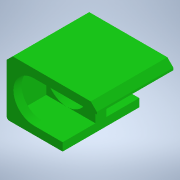
# Autodesk Inventor part: Y-linear bearing shroud secondary
Saved by Autodesk Inventor 2020 (Build 240168000, 168)
## iProperties
Created: 2021-02-25
Part Number: Y-linear bearing shroud secondary
Material: ABS Plastic
Document SubType Name: Modeling
Designer: AOB
Mass: 6.31823 g
Surface Area: 48.6976 cm^2
Volume: 5.96059 cm^3
Density: 1.06 g/cm^3
Appearance: Dark Green
Author: AOB
Autodesk Inventor part; units mm, degrees
ref_plane "YZ Plane" through (0, 0, 0) normal (1, 0, 0) x (0, 1, 0)
ref_plane "XZ Plane" through (0, 0, 0) normal (0, 1, 0) x (-1, 0, 0)
ref_plane "XY Plane" through (0, 0, 0) normal (0, 0, 1) x (1, 0, 0)
sketch "Sketch1" plane through (0, 0, 0) normal (0, 0, 1) x (1, 0, 0)
  line L0 (-9.0445, -10.4807) -> (0.0261, -10.458)
  line L1 (-10, 8.3388) -> (-10, 0)
  line L2 (-10, 0) -> (-9.9763, -9.4855)
  line L3 (-7.782, 10.5568) -> (20.782, 10.5568)
  line L4 (23, 8.3389) -> (23, 7.5575)
  line L5 (20.782, 10.5568) -> (23, 8.3389)
  line L6 (-7.782, 10.5568) -> (-10, 8.3388)
  arc A0 (-9.9763, -9.4855) -> (-8.9738, -10.483) centre (-8.9763, -9.483) ccw
  line L7 (23, 7.5575) -> (5, 7.5125)
  arc A1 (-0.0187, 7.5) -> (0.0187, -7.5) centre (0, 0) ccw
  line L8 (5, 7.5125) -> (-0.0187, 7.5)
  line L9 (0.0261, -10.458) -> (7.5, -10.458)
  line L10 (7.5, 0.0187) -> (10.5, 0.0187) construction
  line L11 (10.5, -10.458) -> (7.5, -10.458)
  line L12 (0.0187, -7.5) -> (10.5, -7.5)
  line L13 (10.5, -7.5) -> (10.5, -10.458)
  line L14 (-8.782, 10.5568) -> (-7.782, 10.5568)
  point P0 (-10.0264, 10.5568)
  point P1 (20.782, 10.5568)
  point P2 (23, 10.5568)
  point P3 (-10, 10.5568)
  dimension "d0" = 2.218
  dimension "d40" = 1
  constraints: 30 end point, 5 point on circle, 5 point on line, 3 horizontal, 3 perpendicular, 2 centre point, 2 tangent, 1 parallel, 1 vertical
  measures "d0" distance of L3.start point (-10, 10.557)
  measures "d40" distance of L3.start L14.start
extrude "Extrusion1" add sketch "Sketch1" along normal blind 3
sketch "Sketch2" plane through (0, 0, 0) normal (0, 0, -1) x (-1, 0, 0)
  line L0 (0.0187, 7.5) -> (-23, 7.5575) projected
  line L1 (-23, 7.5575) -> (-23, 8.3389) projected
  line L2 (-23, 7.5575) -> (-23, 8.3389)
  line L3 (-23, 8.3389) -> (-20.782, 10.5568) projected
  line L4 (-23, 8.3389) -> (-20.782, 10.5568)
  line L5 (-20.782, 10.5568) -> (7.782, 10.5568) projected
  line L6 (-20.782, 10.5568) -> (7.782, 10.5568)
  line L7 (7.782, 10.5568) -> (10, 8.3389)
  line L8 (7.782, 10.5568) -> (10, 8.3388) projected
  line L9 (10, 8.3389) -> (10, -9.4831)
  line L10 (9.0445, -10.4807) -> (-0.0261, -10.458) projected
  line L11 (9.0681, -10.4808) -> (7.5, -10.4768)
  line L12 (-5, 7.5125) -> (-23, 7.5575)
  arc A0 (8.9975, -10.4831) -> (10, -9.4831) centre (9, -9.4831) ccw
  line L13 (-5, 7.5125) -> (7.5, 7.5125)
  arc A1 (-0.0187, -7.5) -> (0.0187, 7.5) centre (0, 0) ccw projected
  line L14 (7.5, 0) -> (7.5, 7.5125)
  line L15 (7.5, -7.5188) -> (7.5, 0)
  line L16 (-0.0187, -7.5) -> (7.5, -7.5188)
  line L17 (-10.5, -7.5) -> (-10.5, -10.458)
  line L18 (-10.5, -7.5) -> (-0.0187, -7.5) projected
  line L19 (-10.5, -7.5) -> (-0.0187, -7.5)
  line L20 (-10.5, -10.458) -> (-0.0261, -10.458)
  point P0 (7.5, -7.5)
  dimension "d3" = 1
  constraints: 27 end point, 7 collinear, 4 point on circle, 3 point on line, 3 tangent, 3 vertical, 2 horizontal, 1 centre point, 1 parallel
  measures "d3" radius of A0
extrude "Extrusion2" add sketch "Sketch2" along normal blind 11 contours L0 L1 L3 L5 L7 L9 A0 L11 L10 L20 L17 L18 L16 L15 L14 L13
ref_plane "Work Plane1" through (0, 0, -11) normal (0, 0, -1) x (-1, 0, 0)
sketch "Sketch4" plane through (0, 0, -11) normal (0, 0, -1) x (-1, 0, 0)
  arc A0 (7.5, 0) -> (0.0187, 7.5) centre (0, 0) ccw
  line L0 (7.5, 7.5125) -> (7.5, -7.5188) projected
  line L1 (7.5, 0) -> (7.5, 7.5125)
  line L2 (7.5, 7.5125) -> (-5, 7.5125) projected
  line L3 (-5, 7.5125) -> (-23, 7.5575) projected
  line L4 (-7.4813, 7.5125) -> (-7.4812, 7.5187)
  arc A1 (-5, 5.5902) -> (-0.0187, -7.5) centre (0, 0) ccw projected
  line L5 (0.0187, 7.5) -> (7.5, 7.5125)
  point P0 (7.5, -10.4768)
  constraints: 6 end point, 2 point on circle, 2 point on line, 1 centre point, 1 coincident, 1 collinear, 1 tangent
extrude "Extrusion4" add sketch "Sketch4" against normal blind 2
mirror "Mirror1" about plane through (0, 0, -11) normal (0, 0, -1) of "Extrusion1", "Extrusion2", "Extrusion4"
sketch "Sketch6" plane through (0, 0, -11) normal (0, 0, -1) x (-1, 0, 0)
  line L0 (-10.5, -7.5) -> (-0.0187, -7.5) projected
  arc A0 (0.0187, 7.5) -> (7.5, -0.0187) centre (0, 0) ccw
  line L1 (-10.5, -10.458) -> (-10.5, -7.5) projected
  line L2 (-0.0187, -7.5) -> (-10.5, -7.5)
  line L3 (-10.5, -7.5) -> (-10.5, 7.5262)
  arc A1 (-0.0187, -7.5) -> (0.0187, 7.5) centre (0, 0) ccw projected
  line L4 (0.0187, 7.5) -> (-23, 7.5575) projected
  line L5 (-10.5, 7.5262) -> (0.0187, 7.5)
  arc A2 (-0.0187, -7.5) -> (0.0187, 7.5) centre (0, 0) ccw projected
  line L6 (7.5, -0.0187) -> (7.4812, -7.5187)
  line L7 (7.4812, -7.5187) -> (-0.0187, -7.5)
  line L8 (-12, 7.53) -> (-12, 0.904) construction
  line L9 (-10.5, 0.8964) -> (-7.4462, 0.8964)
  line L10 (-8.9726, 7.5224) -> (-8.9726, 3.3964) construction
  line L11 (-10.5, 3.3964) -> (-6.6869, 3.3964)
  line L12 (-10.5, 3.3964) -> (-10.5, 5.3964)
  line L13 (-10.5, 5.3964) -> (-5.2085, 5.3964)
  line L14 (-10.5, -1.6036) -> (-10.5, 0.8964)
  line L15 (-5.2085, 5.3964) -> (-5.2085, -5.3964)
  line L16 (-10.5, 0.8964) -> (-10.5, -1.6036)
  line L17 (-10.5, 0.8964) -> (-10.5, -1.6036) construction
  spline S0 degree 1 poles (-10.5, 0.8964) (-10.5, -1.6036) knots 1 1 2 2
  line L18 (-10.5, -1.6036) -> (-7.3266, -1.6036)
  point P0 (-10.5, 7.5262)
  dimension "d26" = 6.626
  dimension "d27" = 4.126
  dimension "d28" = 2
  dimension "d35" = 2.5
  dimension "d41" = 2.5
  constraints: 30 end point, 10 point on circle, 6 point on line, 5 horizontal, 4 collinear, 4 tangent, 3 vertical, 2 perpendicular, 1 centre point, 1 coincident, 3 other
  measures "d26" distance of L8.start L8.end
  measures "d27" distance of L10.start L10.end
  measures "d28" distance of L11.start L12.end
  measures "d35" distance of L9.start L14.start
  measures "d41" distance between parallel lines of L9 L11
revolve "Revolution1" add sketch "Sketch6" angle 360 about axis through (10.5, 0.8964, -11) along (-1, 0, 0) contours A0 L11 L3 L13
extrude "Extrusion3" cut sketch "Sketch6" against normal mid plane 11 contours A0 L15
extrude "Extrusion5" add sketch "Sketch6" along normal mid plane 4 contours L3 L18 A0 L0 | A0 L6 L7 | L13 L3 L4 A0 | A0 L11 L3 L13
body "Solid1"
